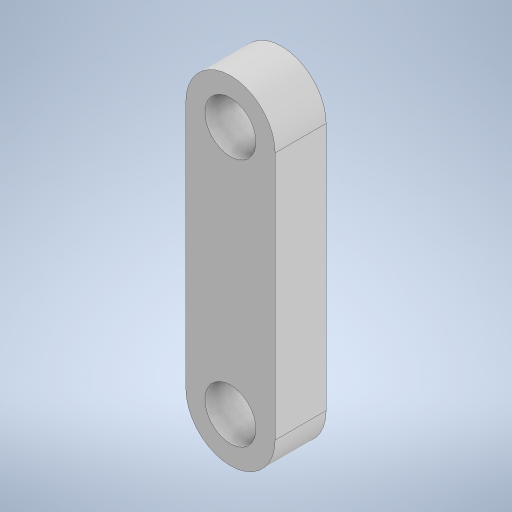
# Autodesk Inventor part: Hebel
Saved by Autodesk Inventor 2024 (Build 280153000, 153)
## iProperties
Created: 2023-05-12
Part Number: Hebel
Material: Generic
Document SubType Name: Modeling
Designer: Raj
Density: 1 g/cm^3
Appearance: Default
Author: Raj
Autodesk Inventor part; units mm, degrees
ref_plane "YZ Plane" through (0, 0, 0) normal (1, 0, 0) x (0, 1, 0)
ref_plane "XZ Plane" through (0, 0, 0) normal (0, 1, 0) x (-1, 0, 0)
ref_plane "XY Plane" through (0, 0, 0) normal (0, 0, 1) x (1, 0, 0)
sketch "Sketch1" plane through (0, 0, 0) normal (0, 1, 0) x (-1, 0, 0)
  line L0 (0, 19.5) -> (0, -19.5) construction
  line L1 (-7, 19.5) -> (-7, -19.5)
  line L2 (7, -19.5) -> (7, 19.5)
  arc A0 (7, 19.5) -> (-7, 19.5) centre (0, 19.5) ccw
  arc A1 (-7, -19.5) -> (7, -19.5) centre (0, -19.5) ccw
  circle A2 centre (0, 19.5) radius 4
  circle A3 centre (0, -19.5) radius 4
  point P0 (0, 0)
  point P1 (0, 0)
  dimension "d0" = 14
  dimension "d1" = 39
  dimension "d3" = 0
  dimension "d4" = 0
  dimension "d5" = 8
  dimension "d6" = 8
  constraints: 8 end point, 4 centre point, 4 point on circle, 4 tangent, 2 coincident, 1 midpoint, 1 parallel, 1 vertical
  measures "d0" diameter of A1
  measures "d1" distance of L0.end L0.start
  measures "d3" distance of point (0, 0) point (0, 0)
  measures "d4" distance of point (0, 0) point (0, 0)
  measures "d5" diameter of A2
  measures "d6" diameter of A3
extrude "Extrusion1" add sketch "Sketch1" along normal blind 8
body "Solid1"
